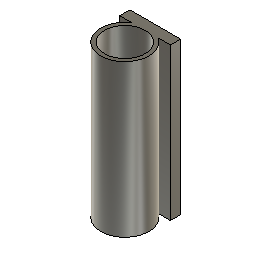
syringe holder (Autodesk Fusion 360 design; units mm, degrees)
Autodesk Fusion 360 part; units mm, degrees
sketch "Sketch1" plane through (0, 0, 0) normal (0, 0, 1) x (1, 0, 0)
  circle A0 centre (0, 0) radius 8
  circle A1 centre (0, 0) radius 9.5
  line L0 (-10, 8) -> (10, 8)
  line L1 (10, 8) -> (10, 12)
  line L2 (10, 12) -> (-10, 12)
  line L3 (-10, 12) -> (-10, 8)
  dimension "d1" = 16
  dimension "d2" = 19
  dimension "d3" = 20
  constraint coincident A0.centre A1.centre
  constraint concentric A0 A1
  constraint horizontal L0
  constraint vertical L1
  constraint horizontal L2
  constraint vertical L3
  measures "d1" diameter of A0
  measures "d2" diameter of A1
  measures "d3" distance of L0.start L0.end
extrude "Extrude1" add sketch "Sketch1" along normal blind 60
